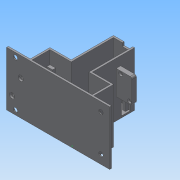
# Autodesk Inventor part: Caja zapato ZOWI DER 2.1
Saved by Autodesk Inventor 2015 (Build 190159000, 159)
## iProperties
Created: 2015-07-30
Part Number: Caja zapato ZOWI DER 2.1
Material: Generic
Document SubType Name: Modeling
Designer: pc
Density: 1 g/cm^3
Appearance: Default
Author: pc
Autodesk Inventor part; units mm, degrees
ref_plane "YZ Plane" through (0, 0, 0) normal (1, 0, 0) x (0, 1, 0)
ref_plane "XZ Plane" through (0, 0, 0) normal (0, 1, 0) x (-1, 0, 0)
ref_plane "XY Plane" through (0, 0, 0) normal (0, 0, 1) x (1, 0, 0)
sketch "Sketch1" plane through (0, 0, 0) normal (0, 0, 1) x (1, 0, 0)
  line L0 (-50.101, 0.6354) -> (-50.101, 25.1354)
  line L1 (-50.101, 25.1354) -> (-25.801, 25.1354)
  line L2 (-25.801, 25.1354) -> (-25.801, 73.4354)
  line L3 (-25.801, 73.4354) -> (-1.601, 73.4354)
  line L4 (-1.601, 73.4354) -> (-1.601, 25.1354)
  line L5 (-1.601, 25.1354) -> (22.699, 25.1354)
  line L6 (22.699, 25.1354) -> (22.699, 0.6354)
  line L7 (22.699, 0.6354) -> (-50.101, 0.6354)
  line L8 (-23.801, 71.4354) -> (-23.801, 23.1354)
  line L9 (-23.801, 23.1354) -> (-48.101, 23.1354)
  line L10 (-48.101, 23.1354) -> (-48.101, 2.6354)
  line L11 (-48.101, 2.6354) -> (20.699, 2.6354)
  line L12 (20.699, 2.6354) -> (20.699, 23.1354)
  line L13 (20.699, 23.1354) -> (-3.601, 23.1354)
  line L14 (-3.601, 23.1354) -> (-3.601, 71.4354)
  line L15 (-3.601, 71.4354) -> (-23.801, 71.4354)
  line L16 (-13.701, 71.4354) -> (-13.701, 50.8657) construction
  line L17 (-13.701, 2.6354) -> (-13.701, -4.6342) construction
  point P0 (0, 0)
  dimension "d1" = 20.2
  dimension "d2" = 2
  dimension "d3" = 20.5
  dimension "d4" = 68.8
  dimension "d6" = 68.8
  constraints: 36 end point, 12 perpendicular, 3 vertical, 2 midpoint, 2 point on line, 1 collinear, 7 other
  measures "d1" distance between parallel lines of L14 L8
  measures "d2" distance between parallel lines of L15 L3
  measures "d3" distance of L11.end L12.end
  measures "d4" distance between parallel lines of L11 L15
  measures "d6" distance between parallel lines of L12 L10
extrude "Extrusion1" add sketch "Sketch1" along normal blind 60
sketch "Sketch2" plane through (0, 0, 0) normal (0, 0, -1) x (-1, 0, 0)
  line L0 (1.601, 73.4354) -> (1.601, 25.1354) projected
  line L1 (25.801, 73.4354) -> (1.601, 73.4354) projected
  line L2 (25.801, 25.1354) -> (25.801, 73.4354) projected
  line L3 (50.101, 25.1354) -> (25.801, 25.1354) projected
  line L4 (50.101, 0.6354) -> (50.101, 25.1354) projected
  line L5 (-22.699, 0.6354) -> (50.101, 0.6354) projected
  line L6 (-22.699, 25.1354) -> (-22.699, 0.6354) projected
  line L7 (1.601, 25.1354) -> (-22.699, 25.1354) projected
  point P0 (0, 0)
extrude "Extrusion2" add sketch "Sketch2" along normal blind 2
sketch "Sketch3" plane through (0, 0, 0) normal (0, 0, 1) x (1, 0, 0)
  line L0 (-3.601, 71.4354) -> (-7.101, 71.4354)
  line L1 (-7.101, 71.4354) -> (-7.101, 64.9354)
  line L2 (-7.101, 64.9354) -> (-3.601, 64.9354)
  line L3 (-3.601, 64.9354) -> (-3.601, 71.4354)
  line L4 (-48.101, 23.1354) -> (-41.601, 23.1354)
  line L5 (-41.601, 23.1354) -> (-41.601, 19.6354)
  line L6 (-41.601, 19.6354) -> (-48.101, 19.6354)
  line L7 (-48.101, 19.6354) -> (-48.101, 23.1354)
  point P0 (0, 0)
  dimension "d15" = 3.5
  dimension "d16" = 6.5
  dimension "d157" = 6.5
  dimension "d158" = 3.5
  constraints: 16 end point, 4 parallel, 2 horizontal, 2 perpendicular
  measures "d15" distance of L1.end L2.end
  measures "d16" distance of L2.end L0.start
  measures "d157" distance of L5.end L6.end
  measures "d158" distance of L4.end L5.end
extrude "Extrusion3" add sketch "Sketch3" along normal blind 45
sketch "Sketch8" plane through (-25.801, 73.4354, 60) normal (0, 1, 0) x (1, 0, 0)
  line L0 (22.2, 60) -> (22.2, 0) projected
  line L1 (12.2, -0.1913) -> (22.2, -0.1913)
  line L2 (22.2, -0.1913) -> (22.2, 3.8087)
  line L3 (22.2, 3.8087) -> (12.2, 3.8087)
  line L4 (12.2, 3.8087) -> (12.2, -0.1913)
  point P0 (25.801, 60)
  dimension "d41" = 4
  dimension "d42" = 10
  constraints: 8 end point, 2 parallel, 1 horizontal, 1 perpendicular, 1 point on line
  measures "d41" distance of L3.end L1.start
  measures "d42" distance of L2.end L3.end
extrude "Extrusion8" cut sketch "Sketch8" against normal blind 2
sketch "Sketch14" plane through (-50.101, 0.6354, 60) normal (0, -1, 0) x (1, 0, 0)
  line L0 (0, 0) -> (-25, 0)
  line L1 (-25, 0) -> (-25, -62)
  line L2 (-25, -62) -> (0, -62)
  line L3 (0, -62) -> (0, 0)
  line L4 (0, -62) -> (0, 0) projected
  line L5 (0, -31) -> (-8.3028, -31) construction
  line L6 (-25, -31) -> (-20.8134, -31) construction
  circle A0 centre (-15, -5) radius 2.5
  line L7 (72.8, -62) -> (92.8, -62)
  line L8 (92.8, -62) -> (92.8, 0)
  line L9 (92.8, 0) -> (72.8, 0)
  line L10 (72.8, 0) -> (72.8, -62)
  line L11 (72.8, 0) -> (48.5, 0) projected
  circle A1 centre (82.8, -10) radius 2.5
  circle A2 centre (-15, -57) radius 2.5
  circle A3 centre (82.8, -52) radius 2.5
  point P0 (50.101, -60)
  dimension "d81" = 62
  dimension "d82" = 25
  dimension "d83" = 5
  dimension "d89" = 5
  dimension "d90" = 10
  dimension "d150" = 5
  dimension "d151" = 10
  dimension "d152" = 10
  dimension "d153" = 20
  dimension "d159" = 5
  dimension "d160" = 5
  dimension "d161" = 5
  dimension "d162" = 10
  dimension "d163" = 10
  dimension "d164" = 10
  constraints: 20 end point, 4 centre point, 4 horizontal, 4 parallel, 3 collinear, 2 midpoint, 2 perpendicular
  measures "d81" distance of L0.end L1.end
  measures "d82" distance of L0.start L0.end
  measures "d83" diameter of A0
  measures "d89" distance from line of L0 A0.centre
  measures "d90" distance from line of L1 A0.centre
  measures "d150" diameter of A1
  measures "d151" distance from line of L10 A1.centre
  measures "d152" distance from line of L9 A1.centre
  measures "d153" distance of L8.end L9.end
  measures "d159" diameter of A2
  measures "d160" diameter of A3
  measures "d161" distance from line of L2 A2.centre
  measures "d162" distance from line of L1 A2.centre
  measures "d163" distance from line of L7 A3.centre
  measures "d164" distance from line of L8 A3.centre
extrude "Extrusion14" add sketch "Sketch14" against normal blind 2
chamfer "Chamfer1" distance 1 angle 45 4 edges at (-67.601, 2.6354, 55) (-67.601, 2.6354, 3) (30.199, 2.6354, 8) (30.199, 2.6354, 50)
sketch "Sketch15" plane through (-50.101, 2.6354, 60) normal (0, 1, 0) x (1, 0, 0)
  line L0 (-6, 47.5876) -> (-22, 47.5876)
  line L1 (-22, 47.5876) -> (-22, 19.5876)
  line L2 (-22, 19.5876) -> (-6, 19.5876)
  line L3 (-6, 19.5876) -> (-6, 47.5876)
  line L4 (0, 0) -> (0, 62) projected
  point P0 (50.101, 60)
  dimension "d91" = 16
  dimension "d92" = 28
  dimension "d93" = 6
  constraints: 8 end point, 2 parallel, 1 horizontal, 1 perpendicular
  measures "d91" distance of L0.start L0.end
  measures "d92" distance between parallel lines of L2 L0
  measures "d93" distance between parallel lines of L4 L3
extrude "Extrusion15" add sketch "Sketch15" along normal blind 2
sketch "Sketch16" plane through (-50.101, 0.6354, 60) normal (-1, 0, 0) x (0, 0, 1)
  line L0 (-47.5876, 4) -> (-19.5876, 4) projected
  line L1 (-59.5876, 15) -> (-29.5876, 15)
  line L2 (-29.5876, 15) -> (-29.5876, 5)
  line L3 (-29.5876, 5) -> (-59.5876, 5)
  line L4 (-59.5876, 5) -> (-59.5876, 15)
  line L5 (-47.5876, 2) -> (-47.5876, 4) projected
  point P0 (-60, -0.6354)
  dimension "d96" = 18
  dimension "d97" = 30
  dimension "d99" = 1
  dimension "d100" = 10
  constraints: 8 end point, 2 parallel, 1 horizontal, 1 perpendicular
  measures "d96" distance between parallel lines of L2 L5
  measures "d97" distance of L1.start L1.end
  measures "d99" distance between parallel lines of L0 L3
  measures "d100" distance between parallel lines of L1 L3
extrude "Extrusion16" cut sketch "Sketch16" against normal blind 2
sketch "Sketch17" plane through (-50.101, 4.6354, 60) normal (0, 1, 0) x (1, 0, 0)
  circle A0 centre (-19, 44.5876) radius 1.5
  circle A1 centre (-9, 22.5876) radius 1.5
  line L0 (-22, 47.5876) -> (-22, 19.5876) projected
  line L1 (-6, 47.5876) -> (-22, 47.5876) projected
  line L2 (-22, 19.5876) -> (-6, 19.5876) projected
  line L3 (-6, 19.5876) -> (-6, 47.5876) projected
  point P0 (50.101, 60)
  dimension "d103" = 3
  dimension "d104" = 3
  dimension "d105" = 3
  dimension "d106" = 3
  dimension "d107" = 3
  dimension "d108" = 3
  constraints: 2 centre point
  measures "d103" diameter of A1
  measures "d104" diameter of A0
  measures "d105" distance from line of L0 A0.centre
  measures "d106" distance from line of L1 A0.centre
  measures "d107" distance from line of L2 A1.centre
  measures "d108" distance from line of L3 A1.centre
extrude "Extrusion17" cut sketch "Sketch17" against normal blind 4 contours A0 | A1
sketch "Sketch18" plane through (-50.101, 0.6354, 60) normal (0, -1, 0) x (1, 0, 0)
  circle A0 centre (-19, -44.5876) radius 3
  circle A1 centre (-9, -22.5876) radius 3
  circle A2 centre (-19, -44.5876) radius 1.5 projected
  circle A3 centre (-9, -22.5876) radius 1.5 projected
  point P0 (50.101, -60)
  dimension "d111" = 6
  dimension "d112" = 6
  constraints: 2 centre point, 2 concentric
  measures "d111" diameter of A0
  measures "d112" diameter of A1
extrude "Extrusion18" cut sketch "Sketch18" against normal blind 2
sketch "Sketch19" plane through (-1.601, 25.1354, 60) normal (1, 0, 0) x (0, 0, -1)
  line L0 (10, 32.3) -> (38, 32.3)
  line L1 (38, 32.3) -> (38, 27.3)
  line L2 (38, 27.3) -> (10, 27.3)
  line L3 (10, 27.3) -> (10, 32.3)
  line L4 (0, 48.3) -> (62, 48.3) projected
  line L5 (0, 0) -> (0, 48.3) projected
  point P0 (60, -25.1354)
  dimension "d115" = 5
  dimension "d116" = 28
  dimension "d119" = 16
  dimension "d120" = 10
  constraints: 8 end point, 2 parallel, 1 horizontal, 1 perpendicular
  measures "d115" distance of L0.end L1.end
  measures "d116" distance of L0.start L0.end
  measures "d119" distance between parallel lines of L4 L0
  measures "d120" distance between parallel lines of L5 L3
extrude "Extrusion19" add sketch "Sketch19" along normal blind 18
sketch "Sketch20" plane through (-1.601, 57.4354, 50) normal (0, 1, 0) x (1, 0, 0)
  circle A0 centre (15, 25) radius 1.5
  circle A1 centre (5, 3) radius 1.5
  line L0 (0, 28) -> (18, 28) projected
  line L1 (18, 28) -> (18, 0) projected
  line L2 (0, 0) -> (18, 0) projected
  line L3 (0, -10) -> (0, 52) projected
  point P0 (1.601, 50)
  dimension "d121" = 3
  dimension "d122" = 3
  dimension "d123" = 3
  dimension "d124" = 3
  dimension "d125" = 3
  dimension "d126" = 5
  constraints: 2 centre point
  measures "d121" diameter of A0
  measures "d122" diameter of A1
  measures "d123" distance from line of L0 A0.centre
  measures "d124" distance from line of L1 A0.centre
  measures "d125" distance from line of L2 A1.centre
  measures "d126" distance from line of L3 A1.centre
extrude "Extrusion20" cut sketch "Sketch20" against normal blind 10 contours A0 | A1
sketch "Sketch21" plane through (-1.601, 52.4354, 22) normal (0, -1, 0) x (1, 0, 0)
  circle A0 centre (5, 25) radius 2.2
  circle A1 centre (15, 3) radius 2.2
  circle A2 centre (15, 3) radius 1.5 projected
  circle A3 centre (5, 25) radius 1.5 projected
  point P0 (1.601, -22)
  dimension "d129" = 4.4
  dimension "d130" = 4.4
  constraints: 2 centre point, 2 concentric
  measures "d129" diameter of A1
  measures "d130" diameter of A0
extrude "Extrusion21" cut sketch "Sketch21" against normal blind 2
fillet "Fillet4" radius 2 2 edges at (16.399, 54.9354, 50) (16.399, 54.9354, 22)
sketch "Sketch22" plane through (-1.601, 25.1354, 60) normal (1, 0, 0) x (0, 0, -1)
  line L0 (20, 43.3) -> (60, 43.3)
  line L1 (60, 43.3) -> (60, 33.3)
  line L2 (60, 33.3) -> (20, 33.3)
  line L3 (20, 33.3) -> (20, 43.3)
  line L4 (36, 32.3) -> (12, 32.3) projected
  line L5 (10, 32.3) -> (10, 27.3) projected
  point P0 (60, -25.1354)
  dimension "d134" = 1
  dimension "d135" = 10
  dimension "d136" = 40
  dimension "d137" = 10
  constraints: 8 end point, 2 parallel, 1 horizontal, 1 perpendicular
  measures "d134" distance between parallel lines of L4 L2
  measures "d135" distance between parallel lines of L2 L0
  measures "d136" distance between parallel lines of L1 L3
  measures "d137" distance between parallel lines of L5 L3
extrude "Extrusion22" cut sketch "Sketch22" against normal blind 2
sketch "Sketch23" plane through (0, 0, 0) normal (0, 0, 1) x (1, 0, 0)
  line L0 (-48.101, 2.6354) -> (-48.101, 23.1354) projected
  line L1 (-3.601, 73.4354) -> (-3.601, 23.1354) projected
  line L2 (-10.601, 22.0354) -> (-3.601, 22.0354)
  line L3 (-3.601, 22.0354) -> (-3.601, 52.0354)
  line L4 (-3.601, 52.0354) -> (-10.601, 52.0354)
  line L5 (-10.601, 52.0354) -> (-10.601, 22.0354)
  line L6 (-28.701, 23.1354) -> (1.299, 23.1354)
  line L7 (1.299, 23.1354) -> (1.299, 16.1354)
  line L8 (1.299, 16.1354) -> (-28.701, 16.1354)
  line L9 (-28.701, 16.1354) -> (-28.701, 23.1354)
  line L10 (-3.601, 23.1354) -> (20.699, 23.1354) projected
  dimension "d147" = 30
  dimension "d149" = 7
  dimension "d154" = 30
  dimension "d155" = 7
  dimension "d156" = 19.4
  constraints: 16 end point, 4 parallel, 2 collinear, 2 horizontal, 2 perpendicular
  measures "d147" distance of L4.end L2.start
  measures "d149" distance of L3.end L4.end
  measures "d154" distance of L7.end L8.end
  measures "d155" distance of L6.end L7.end
  measures "d156" distance between parallel lines of L0 L9
extrude "Extrusion23" cut sketch "Sketch23" against normal blind 2
sketch "Sketch24" plane through (-75.101, 0.6354, -2) normal (0, -1, 0) x (1, 0, 0)
  point P0 (75.101, 2)
body "Solid1"
